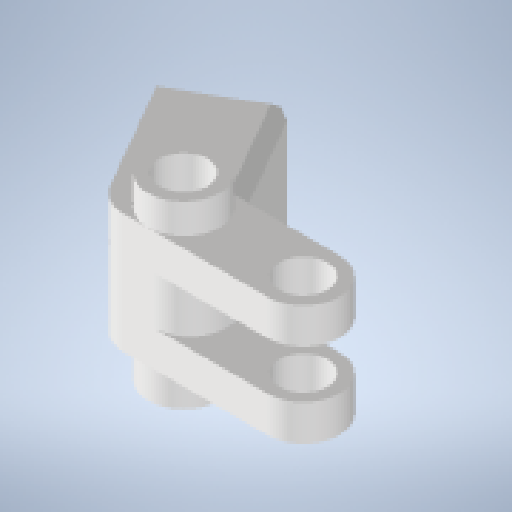
# Autodesk Inventor part: Kniehebel
Saved by Autodesk Inventor 2023.2 (Build 272271030, 271C)
## iProperties
Created: 2023-02-11
Part Number: Kniehebel
Material: Generic
Document SubType Name: Modeling
Designer: Ayush
Density: 1 g/cm^3
Appearance: Default
Author: Ayush
Autodesk Inventor part; units mm, degrees
ref_plane "YZ Plane" through (0, 0, 0) normal (1, 0, 0) x (0, 1, 0)
ref_plane "XZ Plane" through (0, 0, 0) normal (0, 1, 0) x (-1, 0, 0)
sketch "Sketch1" plane through (0, 0, 0) normal (0, 1, 0) x (-1, 0, 0)
  line L0 (0, 0) -> (0, -12)
  circle A0 centre (20, -6) radius 4
  circle A1 centre (0, -6) radius 4
  line L1 (0, -12) -> (15.9795, -12)
  line L2 (15.9795, -12) -> (32.3598, -12) construction
  arc A2 (0, 0) -> (0, -12) centre (0, -6) ccw
  line L3 (15.9795, -12) -> (26.8865, -30.8916)
  line L4 (15.9795, -12) -> (37.7936, -12) construction
  line L5 (26.8865, -30.8916) -> (40.7429, -22.8916)
  line L6 (40.7429, -22.8916) -> (29.2645, -3.0103)
  line L7 (40.7429, -22.8916) -> (77.9933, -22.8916) construction
  line L8 (0, 0) -> (24.0815, 0)
  arc A3 (19.4431, -9.961) -> (19.925, -10.463) centre (24.0503, -6.0207) ccw
  arc A4 (29.2645, -3.0103) -> (24.0815, 0) centre (24.0503, -6.0207) ccw
  arc A5 (19.9091, -1.5614) -> (19.4487, -2.0382) centre (24.0503, -6.0207) ccw
  line L9 (38.9421, -32.689) -> (60.1175, -32.689) construction
  point P0 (0, -6)
  dimension "d1" = 12
  dimension "d4" = 8
  dimension "d5" = 8
  dimension "d9" = 12
  dimension "d14" = 60
  dimension "d15" = 16
  dimension "d16" = 120
  dimension "d21" = 20
  dimension "d22" = 6
  dimension "d23" = 25
  constraints: 20 end point, 10 point on circle, 6 centre point, 6 horizontal, 1 coincident, 1 equal length, 1 midpoint, 1 perpendicular, 1 tangent, 1 vertical
  measures "d1" distance of L0.start L0.end
  measures "d4" diameter of A0
  measures "d5" diameter of A1
  measures "d9" diameter of A2
  measures "d14" angle of L3 L4
  measures "d15" distance of L3.end L5.end
  measures "d16" angle of L7 L6
  measures "d21" distance of A1.centre A0.centre
  measures "d22" vertical distance of L1.end A0.centre
  measures "d23" distance from line of L5 A0.centre
extrude "Extrusion1" add sketch "Sketch1" along normal blind 6 contours L8 A4 L6 L5 L3 L1 L0 A1 | L0 A1 A2
sketch "Sketch2" plane through (0, 6, 0) normal (0, 1, 0) x (1, 0, 0)
  line L0 (-26.8865, 30.8916) -> (-40.7429, 22.8916) projected
  line L1 (-40.7429, 22.8916) -> (-26.8865, 30.8916)
  line L2 (-15.9795, 12) -> (-26.8865, 30.8916) projected
  line L3 (-26.8865, 30.8916) -> (-15.9795, 12)
  line L4 (-40.7429, 22.8916) -> (-29.2645, 3.0103) projected
  line L5 (-40.7429, 22.8916) -> (-29.2585, 3)
  arc A0 (-29.2585, 3) -> (-24.0624, 0) centre (-24.0624, 6) ccw
  line L6 (-24.0815, 0) -> (0, 0) projected
  line L7 (0, 0) -> (-24.0815, 0)
  line L8 (-24.0815, 0) -> (0, 0) projected
  line L9 (0, 12) -> (-15.9795, 12) projected
  line L10 (-15.9795, 12) -> (-12.9795, 12)
  line L11 (-12.9795, 12) -> (-12.9795, 6)
  arc A1 (-18.9795, 0) -> (-12.9795, 6) centre (-18.9795, 6) ccw
  circle A2 centre (0, 6) radius 4 projected
  circle A3 centre (-20, 6) radius 4
  dimension "d26" = 12
  dimension "d27" = 3
  dimension "d28" = 12
  dimension "d30" = 8
  dimension "d32" = 6
  constraints: 12 end point, 4 point on circle, 4 tangent, 3 centre point, 3 collinear, 3 point on line, 1 perpendicular, 1 vertical
  measures "d26" diameter of A0
  measures "d27" distance of L2.start L10.end
  measures "d28" diameter of A1
  measures "d30" diameter of A3
  measures "d32" distance from line of A3.centre L9
ref_plane "Work Plane1" through (0, 10, 0) normal (0, 1, 0) x (1, 0, 0)
mirror "Mirror1" about plane through (0, 10, 0) normal (0, 1, 0) of "Extrusion1"
extrude "Extrusion2" add sketch "Sketch2" along normal blind 8 contours L2 L9 L11 A1 L6 A0 L5 L4 L0
chamfer "Chamfer1" distance 2 angle 45 1 edges at (-33.8147, 20, -26.8916) measured on face at (-29.9672, 20, -21.025)
chamfer "Chamfer2" distance 2 angle 45 1 edges at (-26.8865, 9, -30.8916) measured on face at (-19.2818, 13.3333, -17.7198)
chamfer "Chamfer3" distance 2 angle 45 1 edges at (-40.7429, 9, -22.8916) measured on face at (-36.9168, 8, -16.2645)
chamfer "Chamfer4" distance 2 angle 45 1 edges at (-33.8147, 0, -26.8916) measured on face at (-29.3006, 0, -19.8703)
chamfer "Chamfer5" distance 2 angle 45 1 edges at (-20.933, 20, -20.5798) measured on face at (-19.2818, 6.6667, -17.7198)
chamfer "Chamfer6" distance 2 angle 45 1 edges at (-20.933, 0, -20.5798) measured on face at (-29.3006, 0, -19.8703)
sketch "Sketch3" plane through (-39.0109, 2, -23.8916) normal (-0.5, 0, -0.866) x (-0.866, 0, 0.5)
  line L0 (2, -2) -> (0, 0) projected
  line L1 (-12, 0) -> (-12, 16) projected
  circle A0 centre (-6, 8) radius 6
  line L2 (0, 0) -> (-12, 0) projected
  line L3 (0, 0) -> (0, 16)
  line L4 (-0.9835, 18) -> (-0.9835, 12) projected
  line L5 (-12, 16) -> (0, 16) projected
  line L6 (0, 16) -> (-12, 16)
  line L7 (-12, 16) -> (-12, 0)
  point P0 (-21.8386, -2)
  point P1 (0, 8)
  point P2 (-12, 8)
  dimension "d54" = 12
  constraints: 6 end point, 2 collinear, 1 centre point, 1 parallel
  measures "d54" diameter of A0
extrude "Extrusion3" add sketch "Sketch3" along normal blind 0.01 contours L1 A0 L3 L2 | L1 L5 L3 A0
sketch "Sketch5" plane through (-24.0815, 20, 0) normal (0, 1, 0) x (1, 0, 0)
  line L0 (24.0815, 12) -> (5.7926, 12) projected
  circle A0 centre (4.0815, 6) radius 4
  circle A1 centre (4.0815, 6) radius 6
  point P0 (24.0815, 0)
  dimension "d66" = 8
  dimension "d68" = 12
  constraints: 2 centre point, 1 coincident
  measures "d66" diameter of A0
  measures "d68" diameter of A1
extrude "Extrusion4" add sketch "Sketch5" along normal blind 5
sketch "Sketch6" plane through (0, 0, 0) normal (0, -1, 0) x (1, 0, 0)
  line L0 (0, -12) -> (-18.2889, -12) projected
  circle A0 centre (-20, -6) radius 4
  circle A1 centre (-20, -6) radius 6
  point P0 (0, 0)
  dimension "d73" = 8
  dimension "d75" = 12
  constraints: 2 centre point, 1 coincident
  measures "d73" diameter of A0
  measures "d75" diameter of A1
extrude "Extrusion5" add sketch "Sketch6" along normal blind 5
sketch "Sketch7" plane through (-39.0159, 2, -23.9002) normal (-0.5, 0, -0.866) x (-0.866, 0, 0.5)
  line L0 (-12, 16) -> (-13, 17) projected
  line L1 (2, 18) -> (0, 16) projected
  line L2 (-12, 0) -> (0, 0) projected
  circle A0 centre (-6, 8) radius 6
  point P0 (-21.8386, -2)
  dimension "d78" = 12
  constraints: 1 centre point
  measures "d78" diameter of A0
hole "Hole2" at (-33.8197, 10, -26.9002) direction (0.5, 0, 0.866) diameter 12 depth 16 tip angle 118
thread "Thread1" size "M12x1" class "6H" standard "ANSI Metric M Profile" full length
body "Solid1"
